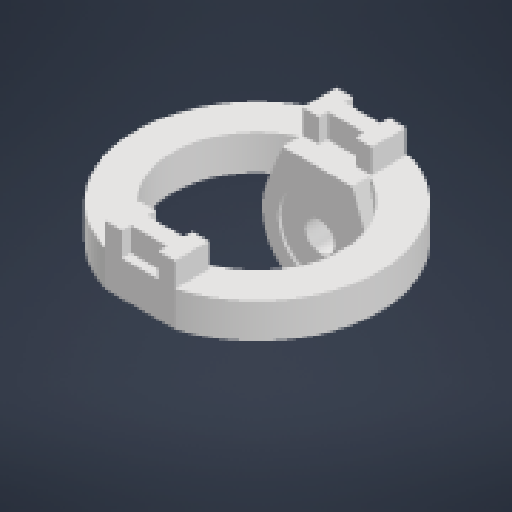
# Autodesk Inventor part: 45angleBase
Saved by Autodesk Inventor 2026 (Build 300175050, 175E)
## iProperties
Created: 2026-04-30
Part Number: 45angleBase
Material: Generic
Document SubType Name: Modeling
Designer: sniel
Density: 1 g/cm^3
Appearance: Default
Author: sniel
Autodesk Inventor part; units mm, degrees
ref_plane "YZ Plane" through (0, 0, 0) normal (1, 0, 0) x (0, 1, 0)
ref_plane "XZ Plane" through (0, 0, 0) normal (0, 1, 0) x (-1, 0, 0)
ref_plane "XY Plane" through (0, 0, 0) normal (0, 0, 1) x (1, 0, 0)
sketch "Sketch1" plane through (0, 0, 0) normal (1, 0, 0) x (0, 1, 0)
  line L0 (0, 22.9155) -> (0, 32.9155)
  line L1 (7, 22.9155) -> (0, 22.9155)
  line L2 (7, 32.9155) -> (7, 22.9155)
  line L3 (7, 32.9155) -> (0, 32.9155)
  line L4 (0, -32.9155) -> (0, -22.9155)
  line L5 (7, -32.9155) -> (0, -32.9155)
  line L6 (7, -22.9155) -> (7, -32.9155)
  line L7 (7, -22.9155) -> (0, -22.9155)
  line L8 (7, 32.9155) -> (6.85, 32.9155)
  line L9 (6.85, 32.9155) -> (6.85, 32.7655)
  line L10 (6.85, 32.7655) -> (7, 32.7655)
  line L11 (7, 32.7655) -> (7, 32.9155)
  line L12 (7, 22.9155) -> (6.85, 22.9155)
  line L13 (6.85, 22.9155) -> (6.85, 23.0655)
  line L14 (6.85, 23.0655) -> (7, 23.0655)
  line L15 (7, 23.0655) -> (7, 22.9155)
  line L16 (7, -22.9155) -> (6.85, -22.9155)
  line L17 (6.85, -22.9155) -> (6.85, -23.0655)
  line L18 (6.85, -23.0655) -> (7, -23.0655)
  line L19 (7, -23.0655) -> (7, -22.9155)
  line L20 (7, -32.9155) -> (6.85, -32.9155)
  line L21 (6.85, -32.9155) -> (6.85, -32.7655)
  line L22 (6.85, -32.7655) -> (7, -32.7655)
  line L23 (7, -32.7655) -> (7, -32.9155)
  line L24 (6.85, 32.7655) -> (0, 32.7655)
  line L25 (0, 32.7655) -> (0, 23.0655)
  line L26 (0, 23.0655) -> (6.85, 23.0655)
  line L27 (6.85, 23.0655) -> (6.85, 32.7655)
  line L28 (6.85, -23.0655) -> (0, -23.0655)
  line L29 (0, -23.0655) -> (0, -32.7655)
  line L30 (0, -32.7655) -> (6.85, -32.7655)
  line L31 (6.85, -32.7655) -> (6.85, -23.0655)
  point P0 (0, -23.0655)
  point P1 (0, 32.7655)
  dimension "d0" = 0.15
  dimension "d1" = 0.15
  dimension "d2" = 0.15
  dimension "d3" = 0.15
  dimension "d4" = 0.15
  dimension "d5" = 0.15
  dimension "d6" = 0.15
  dimension "d7" = 0.15
  constraints: 64 end point, 12 parallel, 6 horizontal, 6 perpendicular, 4 point on line
  measures "d0" distance of L10.end L9.end
  measures "d1" distance of L9.end L8.end
  measures "d2" distance of L13.end L14.end
  measures "d3" distance of L12.end L13.end
  measures "d4" distance of L18.end L17.end
  measures "d5" distance of L17.end L16.end
  measures "d6" distance of L21.end L22.end
  measures "d7" distance of L20.end L21.end
extrude "Extrusion1" add sketch "Sketch1" along normal blind 4.7 contours L0 L24 L27 L26 | L4 L28 L31 L30
sketch "Sketch2" plane through (0, 0, 23.0655) normal (0, -1, 0) x (1, 0, 0)
  line L0 (-58.481, -28.481) -> (-58.481, -18.481) projected
  line L1 (-58.481, -18.481) -> (-48.481, -18.481) projected
  line L2 (-48.481, -18.481) -> (-48.481, -28.481) projected
  line L3 (-48.481, -28.481) -> (-58.481, -28.481) projected
  arc A0 (-5.25, 39.85) -> (9.85, 24.75) centre (9.85, 39.85) ccw projected
  line L4 (-5.25, 39.85) -> (-11.6285, 39.85) projected
  arc A1 (-15.1285, 39.85) -> (-11.6285, 39.85) centre (-13.3785, 39.85) ccw projected
  line L5 (-15.1285, 39.85) -> (-22.65, 39.85) projected
  line L6 (-22.65, 39.85) -> (-22.65, 34.85) projected
  line L7 (-22.65, 34.85) -> (-20.15, 34.85) projected
  line L8 (-20.15, 34.85) -> (-20.15, 29.85) projected
  line L9 (-20.15, 29.85) -> (-30.15, 29.85) projected
  line L10 (-30.15, 29.85) -> (-30.15, 34.85) projected
  line L11 (-30.15, 34.85) -> (-27.65, 34.85) projected
  line L12 (-27.65, 34.85) -> (-27.65, 39.85) projected
  line L13 (-27.65, 39.85) -> (-42.381, 39.85) projected
  arc A2 (-64.581, 39.85) -> (-42.381, 39.85) centre (-53.481, 39.85) ccw projected
  line L14 (-64.581, 39.85) -> (-78.481, 39.85) projected
  line L15 (-78.481, 39.85) -> (-78.481, 34.85) projected
  line L16 (-78.481, 34.85) -> (-75.981, 34.85) projected
  line L17 (-75.981, 34.85) -> (-75.981, 29.85) projected
  line L18 (-75.981, 29.85) -> (-85.981, 29.85) projected
  line L19 (-85.981, 29.85) -> (-85.981, 34.85) projected
  line L20 (-85.981, 34.85) -> (-83.481, 34.85) projected
  line L21 (-83.481, 34.85) -> (-83.481, 39.85) projected
  line L22 (-83.481, 39.85) -> (-112.3855, 39.85) projected
  arc A3 (-112.3855, 39.85) -> (9.85, -82.3855) centre (9.85, 39.85) ccw projected
  line L23 (9.85, -82.3855) -> (9.85, -53.481) projected
  line L24 (9.85, -53.481) -> (4.85, -53.481) projected
  line L25 (4.85, -53.481) -> (4.85, -55.981) projected
  line L26 (4.85, -55.981) -> (-0.15, -55.981) projected
  line L27 (-0.15, -55.981) -> (-0.15, -45.981) projected
  line L28 (-0.15, -45.981) -> (4.85, -45.981) projected
  line L29 (4.85, -45.981) -> (4.85, -48.481) projected
  line L30 (4.85, -48.481) -> (9.85, -48.481) projected
  line L31 (9.85, -48.481) -> (9.85, -34.581) projected
  arc A4 (9.85, -12.381) -> (9.85, -34.581) centre (9.85, -23.481) ccw projected
  line L32 (9.85, -12.381) -> (9.85, 2.35) projected
  line L33 (9.85, 2.35) -> (4.85, 2.35) projected
  line L34 (4.85, 2.35) -> (4.85, -0.15) projected
  line L35 (4.85, -0.15) -> (-0.15, -0.15) projected
  line L36 (-0.15, -0.15) -> (-0.15, 9.85) projected
  line L37 (-0.15, 9.85) -> (4.85, 9.85) projected
  line L38 (4.85, 9.85) -> (4.85, 7.35) projected
  line L39 (4.85, 7.35) -> (9.85, 7.35) projected
  line L40 (9.85, 7.35) -> (9.85, 14.8715) projected
  arc A5 (9.85, 18.3715) -> (9.85, 14.8715) centre (9.85, 16.6215) ccw projected
  line L41 (9.85, 18.3715) -> (9.85, 24.75) projected
  line L42 (78.181, -28.481) -> (68.181, -28.481) projected
  line L43 (68.181, -28.481) -> (68.181, -18.481) projected
  line L44 (68.181, -18.481) -> (78.181, -18.481) projected
  line L45 (78.181, -18.481) -> (78.181, -28.481) projected
  arc A6 (9.85, 24.75) -> (24.95, 39.85) centre (9.85, 39.85) ccw projected
  line L46 (9.85, 24.75) -> (9.85, 18.3715) projected
  arc A7 (9.85, 14.8715) -> (9.85, 18.3715) centre (9.85, 16.6215) ccw projected
  line L47 (9.85, 14.8715) -> (9.85, 7.35) projected
  line L48 (9.85, 7.35) -> (14.85, 7.35) projected
  line L49 (14.85, 7.35) -> (14.85, 9.85) projected
  line L50 (14.85, 9.85) -> (19.85, 9.85) projected
  line L51 (19.85, 9.85) -> (19.85, -0.15) projected
  line L52 (19.85, -0.15) -> (14.85, -0.15) projected
  line L53 (14.85, -0.15) -> (14.85, 2.35) projected
  line L54 (14.85, 2.35) -> (9.85, 2.35) projected
  line L55 (9.85, 2.35) -> (9.85, -12.381) projected
  arc A8 (9.85, -34.581) -> (9.85, -12.381) centre (9.85, -23.481) ccw projected
  line L56 (9.85, -34.581) -> (9.85, -48.481) projected
  line L57 (9.85, -48.481) -> (14.85, -48.481) projected
  line L58 (14.85, -48.481) -> (14.85, -45.981) projected
  line L59 (14.85, -45.981) -> (19.85, -45.981) projected
  line L60 (19.85, -45.981) -> (19.85, -55.981) projected
  line L61 (19.85, -55.981) -> (14.85, -55.981) projected
  line L62 (14.85, -55.981) -> (14.85, -53.481) projected
  line L63 (14.85, -53.481) -> (9.85, -53.481) projected
  line L64 (9.85, -53.481) -> (9.85, -82.3855) projected
  arc A9 (9.85, -82.3855) -> (132.0855, 39.85) centre (9.85, 39.85) ccw projected
  line L65 (132.0855, 39.85) -> (103.181, 39.85) projected
  line L66 (103.181, 39.85) -> (103.181, 34.85) projected
  line L67 (103.181, 34.85) -> (105.681, 34.85) projected
  line L68 (105.681, 34.85) -> (105.681, 29.85) projected
  line L69 (105.681, 29.85) -> (95.681, 29.85) projected
  line L70 (95.681, 29.85) -> (95.681, 34.85) projected
  line L71 (95.681, 34.85) -> (98.181, 34.85) projected
  line L72 (98.181, 34.85) -> (98.181, 39.85) projected
  line L73 (98.181, 39.85) -> (84.281, 39.85) projected
  arc A10 (62.081, 39.85) -> (84.281, 39.85) centre (73.181, 39.85) ccw projected
  line L74 (62.081, 39.85) -> (47.35, 39.85) projected
  line L75 (47.35, 39.85) -> (47.35, 34.85) projected
  line L76 (47.35, 34.85) -> (49.85, 34.85) projected
  line L77 (49.85, 34.85) -> (49.85, 29.85) projected
  line L78 (49.85, 29.85) -> (39.85, 29.85) projected
  line L79 (39.85, 29.85) -> (39.85, 34.85) projected
  line L80 (39.85, 34.85) -> (42.35, 34.85) projected
  line L81 (42.35, 34.85) -> (42.35, 39.85) projected
  line L82 (42.35, 39.85) -> (34.8285, 39.85) projected
  arc A11 (31.3285, 39.85) -> (34.8285, 39.85) centre (33.0785, 39.85) ccw projected
  line L83 (31.3285, 39.85) -> (24.95, 39.85) projected
  line L84 (0, 9.7) -> (0, 0) projected
  line L85 (0, 0) -> (4.7, 0) projected
  line L86 (4.7, 9.7) -> (4.7, 0) projected
  line L87 (0, 9.7) -> (4.7, 9.7) projected
  line L88 (0, -46.131) -> (0, -55.831)
  line L89 (0, -55.831) -> (4.7, -55.831)
  line L90 (4.7, -46.131) -> (4.7, -55.831)
  line L91 (0, -46.131) -> (4.7, -46.131)
  line L92 (4.85, -48.481) -> (4.7, -48.481)
  line L93 (4.7, -48.481) -> (4.7, -48.631)
  line L94 (4.7, -48.631) -> (4.85, -48.631)
  line L95 (4.85, -48.631) -> (4.85, -48.481)
  line L96 (14.85, -48.481) -> (15, -48.481)
  line L97 (15, -48.481) -> (15, -48.631)
  line L98 (15, -48.631) -> (14.85, -48.631)
  line L99 (14.85, -48.631) -> (14.85, -48.481)
  line L100 (14.85, -55.981) -> (15, -55.981)
  line L101 (15, -55.981) -> (15, -55.831)
  line L102 (15, -55.831) -> (14.85, -55.831)
  line L103 (14.85, -55.831) -> (14.85, -55.981)
  line L104 (19.85, -45.981) -> (19.7, -45.981)
  line L105 (19.7, -45.981) -> (19.7, -46.131)
  line L106 (19.7, -46.131) -> (19.85, -46.131)
  line L107 (19.85, -46.131) -> (19.85, -45.981)
  line L108 (19.7, -46.131) -> (15, -46.131)
  line L109 (15, -46.131) -> (15, -55.831)
  line L110 (15, -55.831) -> (19.7, -55.831)
  line L111 (19.7, -55.831) -> (19.7, -46.131)
  line L112 (4.85, -53.481) -> (4.7, -53.481)
  line L113 (4.7, -53.481) -> (4.7, -53.331)
  line L114 (4.7, -53.331) -> (4.85, -53.331)
  line L115 (4.85, -53.331) -> (4.85, -53.481)
  line L116 (4.7, -53.331) -> (15, -53.331)
  line L117 (15, -53.331) -> (15, -48.631)
  line L118 (15, -48.631) -> (4.7, -48.631)
  line L119 (4.7, -48.631) -> (4.7, -53.331)
  line L120 (4.85, 7.35) -> (4.7, 7.35)
  line L121 (4.7, 7.35) -> (4.7, 7.2)
  line L122 (4.7, 7.2) -> (4.85, 7.2)
  line L123 (4.85, 7.2) -> (4.85, 7.35)
  line L124 (19.7, 9.7) -> (15, 9.7)
  line L125 (15, 9.7) -> (15, 0)
  line L126 (15, 0) -> (19.7, 0)
  line L127 (19.7, 0) -> (19.7, 9.7)
  line L128 (4.7, 2.5) -> (15, 2.5)
  line L129 (15, 2.5) -> (15, 7.2)
  line L130 (15, 7.2) -> (4.7, 7.2)
  point P0 (0, -23.0655)
  point P1 (4.85, 7.2)
  point P2 (4.7, 7.2)
  point P3 (15, -28.3797)
  point P4 (4.7, -48.631)
  dimension "d10" = 0.15
  dimension "d11" = 0.15
  dimension "d12" = 0.15
  dimension "d13" = 0.15
  dimension "d14" = 0.15
  dimension "d15" = 0.15
  dimension "d16" = 0.15
  dimension "d17" = 0.15
  dimension "d18" = 0.15
  dimension "d19" = 0.15
  dimension "d20" = 0.15
  dimension "d21" = 0.15
  constraints: 86 end point, 19 parallel, 10 horizontal, 10 perpendicular
  measures "d10" distance of L94.end L93.end
  measures "d11" distance of L93.end L92.end
  measures "d12" distance of L97.end L98.end
  measures "d13" distance of L96.end L97.end
  measures "d14" distance of L102.end L101.end
  measures "d15" distance of L101.end L100.end
  measures "d16" distance of L106.end L105.end
  measures "d17" distance of L105.end L104.end
  measures "d18" distance of L113.end L114.end
  measures "d19" distance of L112.end L113.end
  measures "d20" distance of L122.end L121.end
  measures "d21" distance of L121.end L120.end
extrude "Extrusion2" add sketch "Sketch2" against normal blind 6.85 contours L130 L125 L128 L86 L122 | L125 L124 L127 L126 | L118 L98 L109 L116 L114 L90 L94 | L109 L108 L111 L110 L97
sketch "Sketch3" plane through (0, 0, -32.7655) normal (0, -1, 0) x (1, 0, 0)
  line L0 (0, 9.7) -> (0, 0)
  line L1 (0, 0) -> (4.7, 0)
  line L2 (4.7, 2.5) -> (4.7, 0)
  line L3 (4.7, 2.5) -> (15, 2.5)
  line L4 (15, 2.5) -> (15, 0)
  line L5 (15, 0) -> (19.7, 0)
  line L6 (19.7, 0) -> (19.7, 9.7)
  line L7 (19.7, 9.7) -> (15, 9.7)
  line L8 (15, 9.7) -> (15, 7.2)
  line L9 (15, 7.2) -> (4.7, 7.2)
  line L10 (4.7, 9.7) -> (4.7, 7.2)
  line L11 (0, 9.7) -> (4.7, 9.7)
  line L12 (19.7, 7.2) -> (0, 7.2)
  line L13 (0, 7.2) -> (0, 2.5)
  line L14 (0, 2.5) -> (19.7, 2.5)
  line L15 (19.7, 2.5) -> (19.7, 7.2)
  point P0 (0, 32.7655)
  constraints: 32 end point, 2 parallel, 2 point on line, 1 horizontal, 1 perpendicular
extrude "Extrusion3" add sketch "Sketch3" along normal blind 30 contours L12 L9 L6 L14 L3 L0
sketch "Sketch4" plane through (15, 6.85, -30.2655) normal (0, 0, -1) x (-1, 0, 0)
  ellipse E0 centre (5.1856, -24.5471) end of major axis (5.1856, -28.5471) minor radius 4 (6.6856, -28.2552) -> (6.6856, -20.839) ccw projected
  circle A0 centre (5.1856, -24.5471) radius 11.1
  line L0 (15, -6.85) -> (15, -36.85) projected
  circle A1 centre (5.1856, -24.5471) radius 15.738
  line L1 (-4.7, -6.85) -> (-4.7, -36.85) projected
  line L2 (-4.7, -6.85) -> (-9.4328, -18.717)
  line L3 (15, -6.85) -> (19.7735, -18.6414)
  line L4 (15, -6.85) -> (-4.7, -6.85)
  point P0 (-4.7, -19.4988)
  point P1 (15, -19.3618)
  dimension "d26" = 22.2
  constraints: 6 end point, 3 point on circle, 2 centre point, 2 coincident, 2 tangent, 1 perpendicular, 1 other
  measures "d26" diameter of A0
extrude "Extrusion4" add sketch "Sketch4" against normal up to surface (4.7 mm away) contours A0 L0 | A0 L0 A1 | L0 A0 L1 | L0 A1 L1 A0 | L1 A0 | A0 L1 A1 | L0 L3 A1 | A1 L2 L1 picked at (-2.5391, -36.3696)
sketch "Sketch5" plane through (15, 6.85, -30.2655) normal (0, 0, -1) x (-1, 0, 0)
  arc A0 (-4.6288, -36.85) -> (19.7735, -18.6414) centre (5.1856, -24.5471) ccw projected
  circle A1 centre (5.1856, -24.5471) radius 11.1
  point P0 (15, -6.85)
  dimension "d29" = 22.2
  constraints: 1 centre point, 1 coincident
  measures "d29" diameter of A1
extrude "Extrusion5" cut sketch "Sketch5" against normal blind 10
sketch "Sketch6" plane through (4.7, 6.85, -25.5655) normal (0, 0, 1) x (1, 0, 0)
  circle A0 centre (5.1144, -24.5471) radius 11.1 projected
  line L0 (15, -36.85) -> (14.9288, -36.85) projected
  line L1 (15, -36.7929) -> (15, -36.85) projected
  arc A1 (15, -36.7929) -> (19.7328, -18.717) centre (5.1144, -24.5471) ccw projected
  line L2 (19.7328, -18.717) -> (15, -6.85) projected
  line L3 (10.3, -6.85) -> (15, -6.85) projected
  line L4 (10.3, -6.85) -> (10.3, 0) projected
  line L5 (0, 0) -> (10.3, 0) projected
  line L6 (0, -6.85) -> (0, 0) projected
  line L7 (-4.7, -6.85) -> (0, -6.85) projected
  line L8 (-4.7, -6.85) -> (-9.4735, -18.6414) projected
  arc A2 (-9.4735, -18.6414) -> (14.9288, -36.85) centre (5.1144, -24.5471) ccw projected
  line L9 (0, -6.85) -> (-4.7, -6.85) projected
  line L10 (0, -6.85) -> (10.3, -6.85)
  constraints: 2 end point, 1 collinear
extrude "Extrusion6" add sketch "Sketch6" along normal blind 8.119 contours L0 A2 L8 L7 L10 L3 L2 A1 L1
sketch "Sketch7" plane through (15, 6.85, -30.2655) normal (0, 0, -1) x (-1, 0, 0)
  circle A0 centre (5.1856, -24.5471) radius 11.1 projected
  circle A1 centre (5.1856, -24.5471) radius 4.1
  point P0 (15, -6.85)
  dimension "d34" = 8.2
  constraints: 1 centre point, 1 coincident
  measures "d34" diameter of A1
extrude "Extrusion7" add sketch "Sketch7" against normal blind 12
sketch "Sketch8" plane through (15, 6.85, -30.2655) normal (0, 0, -1) x (-1, 0, 0)
  circle A0 centre (5.1856, -24.5471) radius 4.1 projected
  line L0 (-4.7, -36.7929) -> (-4.7, -36.85) projected
  line L1 (-4.6288, -36.85) -> (-4.7, -36.85) projected
  arc A1 (-4.6288, -36.85) -> (19.7735, -18.6414) centre (5.1856, -24.5471) ccw projected
  line L2 (19.7735, -18.6414) -> (15, -6.85) projected
  line L3 (10.3, -6.85) -> (15, -6.85) projected
  line L4 (10.3, 0) -> (10.3, -6.85) projected
  line L5 (0, 0) -> (10.3, 0) projected
  line L6 (0, -6.85) -> (0, 0) projected
  line L7 (-4.7, -6.85) -> (0, -6.85) projected
  line L8 (-4.7, -6.85) -> (-9.4328, -18.717) projected
  arc A2 (-9.4328, -18.717) -> (-4.7, -36.7929) centre (5.1856, -24.5471) ccw projected
  line L9 (0, -6.85) -> (10.3, -6.85)
  point P0 (15, -6.85)
  constraints: 2 end point, 1 collinear
extrude "Extrusion8" add sketch "Sketch8" along normal up to surface (2.65 mm away) contours A2 L8 L7 L9 L3 L2 A1 L1 L0
sketch "Sketch9" plane through (0, 0, 23.0655) normal (0, -1, 0) x (1, 0, 0)
  line L0 (0, 9.7) -> (0, 0) projected
  line L1 (0, 0) -> (4.7, 0) projected
  line L2 (4.7, 2.5) -> (4.7, 0) projected
  line L3 (4.7, 2.5) -> (15, 2.5) projected
  line L4 (15, 2.5) -> (15, 0) projected
  line L5 (15, 0) -> (19.7, 0) projected
  line L6 (19.7, 0) -> (19.7, 9.7) projected
  line L7 (19.7, 9.7) -> (15, 9.7) projected
  line L8 (15, 9.7) -> (15, 7.2) projected
  line L9 (15, 7.2) -> (4.7, 7.2) projected
  line L10 (4.7, 9.7) -> (4.7, 7.2) projected
  line L11 (0, 9.7) -> (4.7, 9.7) projected
  circle A0 centre (9.85, -23.4777) radius 34.609
  circle A1 centre (9.85, -23.4777) radius 24.0359
  line L12 (5.7144, -55.981) -> (13.9144, -55.981) projected
  line L13 (19.7, -55.981) -> (0, -55.981) projected
  line L14 (24.4328, -55.981) -> (19.7, -55.981) projected
  line L15 (19.7, -55.981) -> (24.4328, -55.981) projected
  line L16 (19.6288, -55.981) -> (19.7, -55.981) projected
  line L17 (-4.7735, -55.981) -> (19.6288, -55.981) projected
  line L18 (0, -55.981) -> (-4.7735, -55.981) projected
  line L19 (19.7, 9.7) -> (0, 9.7)
  point P0 (0, -23.0655)
  point P1 (-2.0375, -55.981)
  point P2 (21.7375, -55.981)
  constraints: 2 end point, 1 coincident, 1 perpendicular, 6 other
extrude "Extrusion9" add sketch "Sketch9" along normal blind 10 contours L11 L10 L9 L8 L7 L6 L5 L4 L3 L2 L1 L0 | L0 L1 A1 L5 L6 A0 L14 L13 L12 L17 | L19 L8 L9 L10 | L2 L3 L4 A1
body "Solid1"
